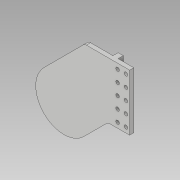
# Autodesk Inventor part: dynamixel_pro_frame_part2
Saved by Autodesk Inventor 2017 (Build 210142000, 142)
## iProperties
Part Number: dynamixel_pro_frame_part2
Material: Aluminium 6061
Document SubType Name: Modeling
Designer: Max
Density: 2.7 g/cm^3
Appearance: Vorgabe
Mass: 57.9575 g
Surface Area: 124.657 cm^2
Volume: 21.4657 cm^3
Author: Max
Autodesk Inventor part; units mm, degrees
ref_plane "YZ Plane" through (0, 0, 0) normal (1, 0, 0) x (0, 1, 0)
ref_plane "XZ Plane" through (0, 0, 0) normal (0, 1, 0) x (-1, 0, 0)
ref_plane "XY Plane" through (0, 0, 0) normal (0, 0, 1) x (1, 0, 0)
sketch "Skizze1" plane through (0, 0, 0) normal (0, 1, 0) x (-1, 0, 0)
  line L0 (20.8162, -27) -> (0, -27)
  line L1 (0, -27) -> (0, 27)
  line L2 (20.8162, -27) -> (43.9081, -50.0919)
  arc A0 (43.9081, -50.0919) -> (82.0919, -11.9081) centre (63, -31) ccw
  line L3 (82.0919, -11.9081) -> (43.1838, 27)
  line L4 (0, 27) -> (43.1838, 27)
  point P0 (0, 0)
  dimension "d0" = 54
  dimension "d40" = 135
  dimension "d42" = 54
  dimension "d43" = 31
  dimension "d47" = 63
  constraints: 10 end point, 2 midpoint, 2 perpendicular, 2 point on circle, 2 tangent, 1 centre point, 1 horizontal, 1 parallel
  measures "d0" distance of L0.end L1.end
  measures "d40" angle of L2 L0
  measures "d42" distance between parallel lines of L3 L2
  measures "d43" vertical distance of point (0, 0) A0.centre
  measures "d47" distance from line of L1 A0.centre
extrude "Extrusion1" add sketch "Skizze1" along normal blind 4
sketch "Skizze3" plane through (0, 4, 0) normal (0, 1, 0) x (1, 0, 0)
  line L0 (0, 0) -> (-17.1865, 0) construction
  line L1 (0, -27) -> (0, 27) construction
  line L2 (0, -27) -> (0, 27) construction
  line L3 (0, 27) -> (-20.8162, 27) construction
  line L4 (-18, -27) -> (0, -27) construction
  line L5 (0, 27) -> (-20.8162, 27) construction
  line L6 (-20.8162, 27) -> (-43.9081, 50.0919) projected
  arc A0 (-43.9081, 50.0919) -> (-82.0919, 11.9081) centre (-63, 31) ccw projected
  line L7 (-82.0919, 11.9081) -> (-43.1838, -27) projected
  line L8 (-43.1838, -27) -> (0, -27) projected
  arc A1 (-43.9081, 50.0919) -> (-82.0919, 11.9081) centre (-63, 31) ccw projected
  circle A2 centre (-63, 31) radius 6
  point P0 (-18, 27)
  dimension "d48" = 12
  constraints: 2 end point, 1 centre point, 1 coincident, 1 horizontal
  measures "d48" diameter of A2
extrude "Extrusion3" [suppressed]
sketch "Skizze5" plane through (0, 4, 0) normal (0, 1, 0) x (1, 0, 0)
  line L0 (0, -27) -> (0, 27) projected
  line L1 (0, 27) -> (-20.8162, 27) projected
  line L2 (-15, -27) -> (-20, -27)
  line L3 (-20, -27) -> (-20, 27)
  line L4 (-20, 27) -> (-15, 27)
  line L5 (-15, 27) -> (-15, -27)
  line L6 (-82.0919, 11.9081) -> (-43.1838, -27) projected
  line L7 (-43.1838, -27) -> (0, -27) projected
  line L8 (-20.8162, 27) -> (-43.9081, 50.0919) projected
  arc A0 (-43.9081, 50.0919) -> (-82.0919, 11.9081) centre (-63, 31) ccw projected
  point P0 (0, 0)
  dimension "d14" = 15
  dimension "d15" = 5
  constraints: 8 end point, 2 parallel, 1 horizontal, 1 perpendicular, 1 point on line
  measures "d14" distance between parallel lines of L5 L0
  measures "d15" distance between parallel lines of L3 L5
extrude "Extrusion4" add sketch "Skizze5" along normal blind 5 contours L2 L3 L1 L5
sketch "Skizze6" plane through (0, 4, 0) normal (0, 1, 0) x (1, 0, 0)
  line L0 (-15, 27) -> (-15, -27) projected
  line L1 (0, -27) -> (0, 27) projected
  line L2 (0, 27) -> (-15, 27) projected
  line L3 (0, 0) -> (67.4565, 0) construction
  line L4 (-15, -27) -> (0, -27) projected
  point P0 (-3.5, 0)
  dimension "d18" = 3.5
  constraints: 2 end point, 1 horizontal, 1 point on line
  measures "d18" distance from line of point (-3.5, 0) L1
hole "Bohrung1" at (-3.5, 4, 0) direction (0, -1, 0) diameter 3.4 end through all clearance for "Inbusschraube ISO 4762" size "M3" standard "ISO"
pattern_linear "Rechteckige Anordnung1" count 5 spacing 11 along (0, 0, -1) count 2 spacing 8 along (-1, 0, 0) of "Bohrung1" first direction both ways yes
sketch "Skizze7" plane through (0, 0, 0) normal (0, -1, 0) x (1, 0, 0)
  circle A0 centre (-63, -31) radius 6
  circle A1 centre (-63, -31) radius 10 construction
  line L0 (-63, -45.6355) -> (-63, -17.0341)
  line L1 (-76.3383, -31) -> (-50.0008, -31)
  circle A2 centre (-63, -31) radius 6 projected
  point P0 (0, 0)
  point P1 (-63, -41)
  point P2 (-73, -31)
  point P3 (-63, -21)
  point P4 (-53, -31)
  dimension "d32" = 20
  constraints: 6 point on line, 4 end point, 4 point on circle, 2 centre point, 2 coincident, 1 horizontal, 1 vertical
  measures "d32" diameter of A1
hole "Bohrung2" [suppressed]
fillet "Rundung1" radius 4 2 edges at (-20.8162, 2, -27) (-43.1838, 2, 27)
sketch "Skizze8" plane through (0, 4, 0) normal (0, 1, 0) x (1, 0, 0)
  arc A0 (-43.9081, 50.0919) -> (-82.0919, 11.9081) centre (-63, 31) ccw projected
  circle A1 centre (-63, 31) radius 6
  circle A2 centre (-63, 31) radius 4
  point P0 (0, 0)
  dimension "d50" = 12
  dimension "d51" = 8
  constraints: 2 centre point, 2 coincident
  measures "d50" diameter of A1
  measures "d51" diameter of A2
extrude "Extrusion5" add sketch "Skizze8" along normal blind 3 contours A1 | A2
extrude "Extrusion6" add sketch "Skizze8" along normal blind 10 contours A2
equation "\"d42\" = d0"
